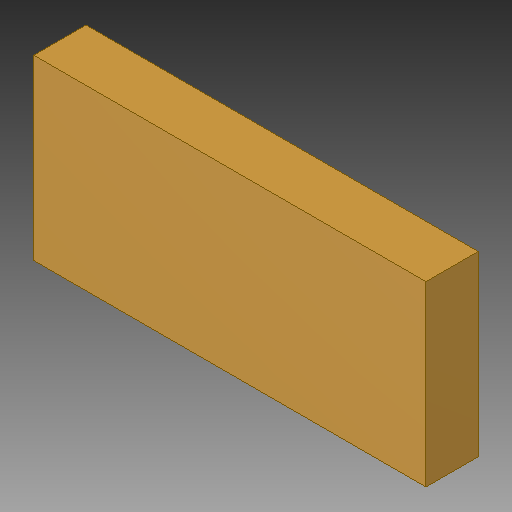
# Autodesk Inventor part: B4B-ZR
Saved by Autodesk Inventor 2019 (Build 230136000, 136)
## iProperties
Created: 2019-10-02
Part Number: B4B-ZR
Material: Generic
Document SubType Name: Modeling
Designer: rybit
Density: 1 g/cm^3
Appearance: B4B-ZR, B4B-ZR
Author: rybit
Autodesk Inventor part; units mm, degrees
ref_plane "YZ Plane" through (0, 0, 0) normal (1, 0, 0) x (0, 1, 0)
ref_plane "XZ Plane" through (0, 0, 0) normal (0, 1, 0) x (-1, 0, 0)
ref_plane "XY Plane" through (0, 0, 0) normal (0, 0, 1) x (1, 0, 0)
sketch "B4B-ZR, B4B-ZR_6" plane through (0, 0, 0) normal (0, 0, 1) x (1, 0, 0)
  line L0 (-3.7516, 1.2) -> (3.7516, 1.2)
  line L1 (3.7516, 1.2) -> (3.7516, -2.2016)
  line L2 (3.7516, -2.2016) -> (-3.7516, -2.2016)
  line L3 (-3.7516, -2.2016) -> (-3.7516, 1.2)
  constraints: 8 end point
extrude "Extrusion1" add sketch "B4B-ZR, B4B-ZR_6" along normal blind 1
body "Solid1"
